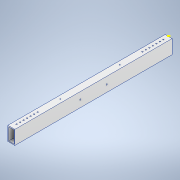
# Autodesk Inventor part: Chassis side 2
Saved by Autodesk Inventor 2022 (Build 260153000, 153)
## iProperties
Created: 2022-11-14
Part Number: Chassis side 2
Material: Aluminum 6061
Document SubType Name: Modeling
Designer: s135320
Mass: 608.37 g
Surface Area: 1428.22 cm^2
Volume: 225.322 cm^3
Density: 2.7 g/cm^3
Appearance: Aluminum - Flat
Author: s135320
Autodesk Inventor part; units mm, degrees
ref_plane "YZ Plane" through (0, 0, 0) normal (1, 0, 0) x (0, 1, 0)
ref_plane "XZ Plane" through (0, 0, 0) normal (0, 1, 0) x (-1, 0, 0)
ref_plane "XY Plane" through (0, 0, 0) normal (0, 0, 1) x (1, 0, 0)
sketch "Sketch1" plane through (0, 0, 0) normal (0, 0, 1) x (1, 0, 0)
  line L0 (-12.7, 25.4) -> (12.7, 25.4)
  line L1 (12.7, 25.4) -> (12.7, -25.4)
  line L2 (12.7, -25.4) -> (-12.7, -25.4)
  line L3 (-12.7, -25.4) -> (-12.7, 25.4)
  line L4 (-12.7, 25.4) -> (12.7, -25.4) construction
  line L5 (12.7, 25.4) -> (-12.7, -25.4) construction
  point P0 (0, 0)
  dimension "d0" = 50.8
  dimension "d1" = 25.4
  constraints: 12 end point, 2 midpoint, 2 parallel, 1 horizontal, 1 perpendicular
  measures "d0" distance of L0.end L1.end
  measures "d1" distance of L0.start L0.end
extrude "Extrusion1" add sketch "Sketch1" along normal blind 571.5
shell "Shell1" thickness 3.175 removed faces 2 at (-4.2333, 8.4667, 571.5) at (-4.2333, 8.4667, 0)
sketch "Sketch2" plane through (-12.7, 25.4, 0) normal (0, 1, 0) x (1, 0, 0)
  line L0 (3.175, -571.5) -> (22.225, -571.5) construction
  line L1 (12.7, -571.5) -> (12.7, -311.4804) construction
  circle A0 centre (12.7, -514.35) radius 2.0701
  circle A1 centre (12.7, -501.65) radius 2.0701
  circle A2 centre (12.7, -488.95) radius 2.0701
  circle A3 centre (12.7, -476.25) radius 2.0701
  circle A4 centre (12.7, -527.05) radius 2.0701
  circle A5 centre (12.7, -514.35) radius 2.0701
  circle A6 centre (12.7, -501.65) radius 2.0701
  circle A7 centre (12.7, -488.95) radius 2.0701
  circle A8 centre (12.7, -539.75) radius 2.0701
  circle A9 centre (12.7, -527.05) radius 2.0701
  circle A10 centre (12.7, -514.35) radius 2.0701
  circle A11 centre (12.7, -501.65) radius 2.0701
  circle A12 centre (12.7, -552.45) radius 2.0701
  circle A13 centre (12.7, -539.75) radius 2.0701
  circle A14 centre (12.7, -527.05) radius 2.0701
  circle A15 centre (12.7, -514.35) radius 2.0701
  line L2 (0, 0) -> (0, -571.5) construction
  line L3 (0, -285.75) -> (25.4, -285.75) construction
  line L4 (25.4, 0) -> (25.4, -571.5) construction
  circle A16 centre (12.7, -57.15) radius 2.0701
  circle A17 centre (12.7, -69.85) radius 2.0701
  circle A18 centre (12.7, -82.55) radius 2.0701
  circle A19 centre (12.7, -95.25) radius 2.0701
  circle A20 centre (12.7, -44.45) radius 2.0701
  circle A21 centre (12.7, -31.75) radius 2.0701
  circle A22 centre (12.7, -19.05) radius 2.0701
  point P0 (12.7, 0)
  dimension "d5" = 4.1402
  dimension "d6" = 57.15
  dimension "d9" = 12.7
  dimension "d12" = 12.7
  constraints: 23 centre point, 7 symmetric about line, 4 end point, 3 midpoint, 3 vertical, 1 point on line, 37 other
  measures "d5" diameter of A0
  measures "d6" distance from line of A0.centre L0
  measures "d9" distance of A0.centre A1.centre
  measures "d12" distance of A0.centre A4.centre
extrude "Extrusion2" cut sketch "Sketch2" against normal through all
sketch "Sketch3" plane through (-12.7, 25.4, 0) normal (0, 1, 0) x (1, 0, 0)
  point P0 (12.7, 0)
sketch "Sketch4" plane through (12.7, -25.4, 0) normal (1, 0, 0) x (0, 0, -1)
  line L0 (-571.5, 0) -> (-571.5, 50.8) construction
  line L1 (-571.5, 25.4) -> (0, 25.4) construction
  line L2 (0, 0) -> (-571.5, 0) construction
  line L3 (-333.375, 36.6437) -> (-238.125, 36.6437) construction
  line L4 (-238.125, 36.6437) -> (-238.125, 14.1563) construction
  line L5 (-238.125, 14.1563) -> (-333.375, 14.1563) construction
  line L6 (-333.375, 14.1563) -> (-333.375, 36.6437) construction
  line L7 (-333.375, 36.6437) -> (-238.125, 14.1563) construction
  line L8 (-238.125, 36.6437) -> (-333.375, 14.1563) construction
  circle A0 centre (-238.125, 25.4) radius 2.0701
  circle A1 centre (-333.375, 25.4) radius 2.0701
  point P0 (-285.75, 25.4)
  dimension "d17" = 95.25
  dimension "d18" = 4.1402
  dimension "d19" = 4.1402
  constraints: 14 end point, 6 midpoint, 3 parallel, 2 centre point, 1 horizontal, 1 perpendicular
  measures "d17" distance of L4.end L5.end
  measures "d18" diameter of A0
  measures "d19" diameter of A1
extrude "Extrusion3" cut sketch "Sketch4" against normal through all
sketch "Sketch5" plane through (-12.7, 25.4, 0) normal (0, 1, 0) x (1, 0, 0)
  line L0 (25.4, -571.5) -> (0, -571.5) construction
  line L1 (12.7, -571.5) -> (12.7, 0) construction
  circle A0 centre (12.7, -393.7) radius 1.5875
  line L2 (25.4, 0) -> (25.4, -571.5) construction
  line L3 (25.4, -285.75) -> (-13.9482, -285.75) construction
  circle A1 centre (12.7, -177.8) radius 1.5875
  dimension "d22" = 3.175
  dimension "d23" = 177.8
  constraints: 4 end point, 2 centre point, 2 midpoint, 1 horizontal, 1 point on line, 1 symmetric about line, 1 vertical, 1 other
  measures "d22" diameter of A0
  measures "d23" distance from line of L0 A0.centre
extrude "Extrusion4" cut sketch "Sketch5" against normal blind 25.4
body "Solid1"
